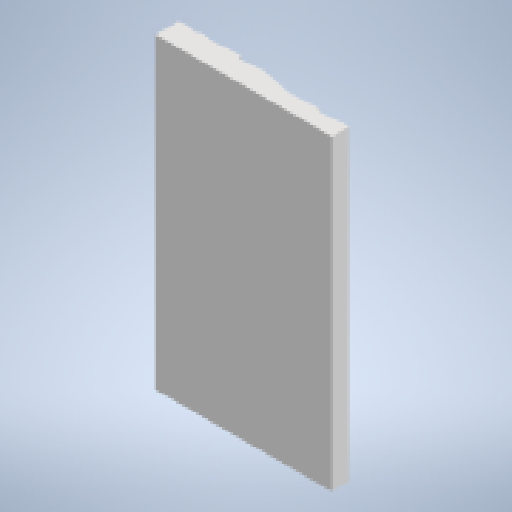
# Autodesk Inventor part: housingPlate
Saved by Autodesk Inventor 2023 (Build 270158000, 158)
## iProperties
Created: 2023-03-11
Part Number: housingPlate
Material: Generic
Document SubType Name: Modeling
Designer: shrey
Density: 1 g/cm^3
Appearance: Default
Author: shrey
Autodesk Inventor part; units mm, degrees
(part 1 of 2)
ref_plane "YZ Plane" through (0, 0, 0) normal (1, 0, 0) x (0, 1, 0)
ref_plane "XZ Plane" through (0, 0, 0) normal (0, 1, 0) x (-1, 0, 0)
ref_plane "XY Plane" through (0, 0, 0) normal (0, 0, 1) x (1, 0, 0)
sketch "Sketch1" plane through (0, 0, 0) normal (0, 0, 1) x (1, 0, 0)
  line L0 (58.171, 304.8) -> (58.171, -304.8) construction
  line L1 (-6.1102, -304.8) -> (58.171, -304.8) projected
  line L2 (-6.1102, 304.8) -> (-6.1102, -304.8) construction
  line L3 (58.171, 304.8) -> (-6.1102, 304.8) projected
  line L4 (-6.1102, 304.8) -> (-6.1102, -304.8) construction
  line L5 (-0.0002, -304.8) -> (-6.1102, -304.8) projected
  line L6 (-0.0002, 304.8) -> (-0.0002, -304.8) construction
  line L7 (-6.1102, 304.8) -> (-0.0002, 304.8) projected
  spline S0 degree 3 poles (-45.7965, -36.1769) (-45.6767, -35.9867) (-45.4969, -35.7016) (-45.2759, -35.3102) (-45.1171, -35.0129) (-44.9666, -34.7113) (-44.8248, -34.4054) (-44.6928, -34.0953) (-44.5714, -33.7808) (-44.4623, -33.4618) (-44.3664, -33.1385) (-44.3039, -32.8646) (-44.2588, -32.6445) (-44.2112, -32.4826) (-44.1468, -32.3266) (-44.0629, -32.1799) (-43.9744, -32.0702) (-43.8945, -31.991) (-43.8269, -31.9405) (-43.7577, -31.8921) (-43.6814, -31.856) (-43.6039, -31.8225) (-43.5218, -31.8027) (-43.4391, -31.786) (-43.3265, -31.782) (-43.1862, -31.7845) (-43.0458, -31.782) (-42.9332, -31.786) (-42.8505, -31.8027) (-42.7684, -31.8225) (-42.6909, -31.856) (-42.6146, -31.8921) (-42.5454, -31.9405) (-42.4778, -31.991) (-42.3979, -32.0702) (-42.3095, -32.1799) (-42.2255, -32.3266) (-42.1611, -32.4826) (-42.1135, -32.6445) (-42.0684, -32.8646) (-42.0059, -33.1385) (-41.91, -33.4618) (-41.8009, -33.7808) (-41.6795, -34.0953) (-41.5475, -34.4054) (-41.4057, -34.7113) (-41.2552, -35.0129) (-41.0964, -35.3102) (-40.8754, -35.7016) (-40.6956, -35.9867) (-40.5758, -36.1769) knots -1.0784 -1.0784 -1.0784 -1.0784 -1.010995 -0.977291 -0.943586 -0.909882 -0.876178 -0.842474 -0.80877 -0.775067 -0.741365 -0.707665 -0.690816 -0.67397 -0.657123 -0.640284 -0.623449 -0.615023 -0.606598 -0.598176 -0.589749 -0.581327 -0.572901 -0.564477 -0.556053 -0.5392 -0.522347 -0.513923 -0.505499 -0.497074 -0.488651 -0.480225 -0.471802 -0.463377 -0.454951 -0.438116 -0.421277 -0.40443 -0.387584 -0.370735 -0.337035 -0.303333 -0.26963 -0.235926 -0.202222 -0.168518 -0.134814 -0.101109 -0.067405 0 0 0 0 construction
  line L8 (-40.5758, -36.1769) -> (-39.5135, -36.1769) construction
  spline S1 degree 3 poles (-39.5135, -36.1769) (-39.3937, -35.9867) (-39.2139, -35.7016) (-38.9929, -35.3102) (-38.8341, -35.0129) (-38.6836, -34.7113) (-38.5418, -34.4054) (-38.4098, -34.0953) (-38.2884, -33.7808) (-38.1793, -33.4618) (-38.0834, -33.1385) (-38.0209, -32.8646) (-37.9758, -32.6445) (-37.9282, -32.4826) (-37.8638, -32.3266) (-37.7799, -32.1799) (-37.6914, -32.0702) (-37.6115, -31.991) (-37.5439, -31.9405) (-37.4747, -31.8921) (-37.3984, -31.856) (-37.3209, -31.8225) (-37.2388, -31.8027) (-37.1561, -31.786) (-37.0435, -31.782) (-36.9032, -31.7845) (-36.7628, -31.782) (-36.6502, -31.786) (-36.5675, -31.8027) (-36.4854, -31.8225) (-36.4079, -31.856) (-36.3316, -31.8921) (-36.2624, -31.9405) (-36.1948, -31.991) (-36.1149, -32.0702) (-36.0265, -32.1799) (-35.9425, -32.3266) (-35.8781, -32.4826) (-35.8305, -32.6445) (-35.7854, -32.8646) (-35.7229, -33.1385) (-35.627, -33.4618) (-35.5179, -33.7808) (-35.3965, -34.0953) (-35.2645, -34.4054) (-35.1227, -34.7113) (-34.9722, -35.0129) (-34.8134, -35.3102) (-34.5924, -35.7016) (-34.4126, -35.9867) (-34.2928, -36.1769) knots -1.0784 -1.0784 -1.0784 -1.0784 -1.010995 -0.977291 -0.943586 -0.909882 -0.876178 -0.842474 -0.80877 -0.775067 -0.741365 -0.707665 -0.690816 -0.67397 -0.657123 -0.640284 -0.623449 -0.615023 -0.606598 -0.598176 -0.589749 -0.581327 -0.572901 -0.564477 -0.556053 -0.5392 -0.522347 -0.513923 -0.505499 -0.497074 -0.488651 -0.480225 -0.471802 -0.463377 -0.454951 -0.438116 -0.421277 -0.40443 -0.387584 -0.370735 -0.337035 -0.303333 -0.26963 -0.235926 -0.202222 -0.168518 -0.134814 -0.101109 -0.067405 0 0 0 0 construction
  line L9 (-34.2928, -36.1769) -> (-33.2305, -36.1769) construction
  spline S2 degree 3 poles (-33.2305, -36.1769) (-33.1107, -35.9867) (-32.9309, -35.7016) (-32.7099, -35.3102) (-32.5511, -35.0129) (-32.4006, -34.7113) (-32.2588, -34.4054) (-32.1268, -34.0953) (-32.0054, -33.7808) (-31.8963, -33.4618) (-31.8004, -33.1385) (-31.7379, -32.8646) (-31.6928, -32.6445) (-31.6452, -32.4826) (-31.5808, -32.3266) (-31.4969, -32.1799) (-31.4084, -32.0702) (-31.3285, -31.991) (-31.2609, -31.9405) (-31.1917, -31.8921) (-31.1154, -31.856) (-31.0379, -31.8225) (-30.9558, -31.8027) (-30.8731, -31.786) (-30.7605, -31.782) (-30.6202, -31.7845) (-30.4798, -31.782) (-30.3672, -31.786) (-30.2845, -31.8027) (-30.2024, -31.8225) (-30.1249, -31.856) (-30.0486, -31.8921) (-29.9794, -31.9405) (-29.9118, -31.991) (-29.8319, -32.0702) (-29.7435, -32.1799) (-29.6595, -32.3266) (-29.5951, -32.4826) (-29.5475, -32.6445) (-29.5024, -32.8646) (-29.4399, -33.1385) (-29.344, -33.4618) (-29.2349, -33.7808) (-29.1135, -34.0953) (-28.9815, -34.4054) (-28.8397, -34.7113) (-28.6892, -35.0129) (-28.5304, -35.3102) (-28.3094, -35.7016) (-28.1296, -35.9867) (-28.0098, -36.1769) knots -1.0784 -1.0784 -1.0784 -1.0784 -1.010995 -0.977291 -0.943586 -0.909882 -0.876178 -0.842474 -0.80877 -0.775067 -0.741365 -0.707665 -0.690816 -0.67397 -0.657123 -0.640284 -0.623449 -0.615023 -0.606598 -0.598176 -0.589749 -0.581327 -0.572901 -0.564477 -0.556053 -0.5392 -0.522347 -0.513923 -0.505499 -0.497074 -0.488651 -0.480225 -0.471802 -0.463377 -0.454951 -0.438116 -0.421277 -0.40443 -0.387584 -0.370735 -0.337035 -0.303333 -0.26963 -0.235926 -0.202222 -0.168518 -0.134814 -0.101109 -0.067405 0 0 0 0 construction
  line L10 (-28.0098, -36.1769) -> (-26.9475, -36.1769) construction
  spline S3 degree 3 poles (-26.9475, -36.1769) (-26.8277, -35.9867) (-26.6479, -35.7016) (-26.4269, -35.3102) (-26.2681, -35.0129) (-26.1176, -34.7113) (-25.9758, -34.4054) (-25.8438, -34.0953) (-25.7224, -33.7808) (-25.6133, -33.4618) (-25.5174, -33.1385) (-25.4549, -32.8646) (-25.4098, -32.6445) (-25.3622, -32.4826) (-25.2978, -32.3266) (-25.2139, -32.1799) (-25.1254, -32.0702) (-25.0455, -31.991) (-24.9779, -31.9405) (-24.9087, -31.8921) (-24.8324, -31.856) (-24.7549, -31.8225) (-24.6728, -31.8027) (-24.5901, -31.786) (-24.4775, -31.782) (-24.3372, -31.7845) (-24.1968, -31.782) (-24.0842, -31.786) (-24.0015, -31.8027) (-23.9194, -31.8225) (-23.8419, -31.856) (-23.7656, -31.8921) (-23.6964, -31.9405) (-23.6288, -31.991) (-23.5489, -32.0702) (-23.4605, -32.1799) (-23.3765, -32.3266) (-23.3121, -32.4826) (-23.2645, -32.6445) (-23.2194, -32.8646) (-23.1569, -33.1385) (-23.061, -33.4618) (-22.9519, -33.7808) (-22.8305, -34.0953) (-22.6985, -34.4054) (-22.5567, -34.7113) (-22.4062, -35.0129) (-22.2474, -35.3102) (-22.0264, -35.7016) (-21.8466, -35.9867) (-21.7268, -36.1769) knots -1.0784 -1.0784 -1.0784 -1.0784 -1.010995 -0.977291 -0.943586 -0.909882 -0.876178 -0.842474 -0.80877 -0.775067 -0.741365 -0.707665 -0.690816 -0.67397 -0.657123 -0.640284 -0.623449 -0.615023 -0.606598 -0.598176 -0.589749 -0.581327 -0.572901 -0.564477 -0.556053 -0.5392 -0.522347 -0.513923 -0.505499 -0.497074 -0.488651 -0.480225 -0.471802 -0.463377 -0.454951 -0.438116 -0.421277 -0.40443 -0.387584 -0.370735 -0.337035 -0.303333 -0.26963 -0.235926 -0.202222 -0.168518 -0.134814 -0.101109 -0.067405 0 0 0 0 construction
  line L11 (-21.7268, -36.1769) -> (-20.6645, -36.1769) construction
  spline S4 degree 3 poles (-20.6645, -36.1769) (-20.5447, -35.9867) (-20.3649, -35.7016) (-20.1439, -35.3102) (-19.9851, -35.0129) (-19.8346, -34.7113) (-19.6928, -34.4054) (-19.5608, -34.0953) (-19.4394, -33.7808) (-19.3303, -33.4618) (-19.2344, -33.1385) (-19.1719, -32.8646) (-19.1268, -32.6445) (-19.0792, -32.4826) (-19.0148, -32.3266) (-18.9309, -32.1799) (-18.8424, -32.0702) (-18.7625, -31.991) (-18.6949, -31.9405) (-18.6257, -31.8921) (-18.5494, -31.856) (-18.4719, -31.8225) (-18.3898, -31.8027) (-18.3071, -31.786) (-18.1945, -31.782) (-18.0542, -31.7845) (-17.9138, -31.782) (-17.8012, -31.786) (-17.7185, -31.8027) (-17.6364, -31.8225) (-17.5589, -31.856) (-17.4826, -31.8921) (-17.4134, -31.9405) (-17.3458, -31.991) (-17.2659, -32.0702) (-17.1775, -32.1799) (-17.0935, -32.3266) (-17.0291, -32.4826) (-16.9815, -32.6445) (-16.9364, -32.8646) (-16.8739, -33.1385) (-16.778, -33.4618) (-16.6689, -33.7808) (-16.5475, -34.0953) (-16.4155, -34.4054) (-16.2737, -34.7113) (-16.1232, -35.0129) (-15.9644, -35.3102) (-15.7434, -35.7016) (-15.5636, -35.9867) (-15.4438, -36.1769) knots -1.0784 -1.0784 -1.0784 -1.0784 -1.010995 -0.977291 -0.943586 -0.909882 -0.876178 -0.842474 -0.80877 -0.775067 -0.741365 -0.707665 -0.690816 -0.67397 -0.657123 -0.640284 -0.623449 -0.615023 -0.606598 -0.598176 -0.589749 -0.581327 -0.572901 -0.564477 -0.556053 -0.5392 -0.522347 -0.513923 -0.505499 -0.497074 -0.488651 -0.480225 -0.471802 -0.463377 -0.454951 -0.438116 -0.421277 -0.40443 -0.387584 -0.370735 -0.337035 -0.303333 -0.26963 -0.235926 -0.202222 -0.168518 -0.134814 -0.101109 -0.067405 0 0 0 0 construction
  line L12 (-15.4438, -36.1769) -> (-14.3815, -36.1769) construction
  spline S5 degree 3 poles (-14.3815, -36.1769) (-14.2617, -35.9867) (-14.0819, -35.7016) (-13.8609, -35.3102) (-13.7021, -35.0129) (-13.5516, -34.7113) (-13.4098, -34.4054) (-13.2778, -34.0953) (-13.1564, -33.7808) (-13.0473, -33.4618) (-12.9514, -33.1385) (-12.8889, -32.8646) (-12.8438, -32.6445) (-12.7962, -32.4826) (-12.7318, -32.3266) (-12.6479, -32.1799) (-12.5594, -32.0702) (-12.4795, -31.991) (-12.4119, -31.9405) (-12.3427, -31.8921) (-12.2664, -31.856) (-12.1889, -31.8225) (-12.1068, -31.8027) (-12.0241, -31.786) (-11.9115, -31.782) (-11.7712, -31.7845) (-11.6308, -31.782) (-11.5182, -31.786) (-11.4355, -31.8027) (-11.3534, -31.8225) (-11.2759, -31.856) (-11.1996, -31.8921) (-11.1304, -31.9405) (-11.0628, -31.991) (-10.9829, -32.0702) (-10.8945, -32.1799) (-10.8105, -32.3266) (-10.7461, -32.4826) (-10.6985, -32.6445) (-10.6534, -32.8646) (-10.5909, -33.1385) (-10.495, -33.4618) (-10.3859, -33.7808) (-10.2645, -34.0953) (-10.1325, -34.4054) (-9.9907, -34.7113) (-9.8402, -35.0129) (-9.6814, -35.3102) (-9.4604, -35.7016) (-9.2806, -35.9867) (-9.1608, -36.1769) knots -1.0784 -1.0784 -1.0784 -1.0784 -1.010995 -0.977291 -0.943586 -0.909882 -0.876178 -0.842474 -0.80877 -0.775067 -0.741365 -0.707665 -0.690816 -0.67397 -0.657123 -0.640284 -0.623449 -0.615023 -0.606598 -0.598176 -0.589749 -0.581327 -0.572901 -0.564477 -0.556053 -0.5392 -0.522347 -0.513923 -0.505499 -0.497074 -0.488651 -0.480225 -0.471802 -0.463377 -0.454951 -0.438116 -0.421277 -0.40443 -0.387584 -0.370735 -0.337035 -0.303333 -0.26963 -0.235926 -0.202222 -0.168518 -0.134814 -0.101109 -0.067405 0 0 0 0 construction
  line L13 (-9.1608, -36.1769) -> (-8.0985, -36.1769) construction
  spline S6 degree 3 poles (-8.0985, -36.1769) (-7.9787, -35.9867) (-7.7989, -35.7016) (-7.5779, -35.3102) (-7.4191, -35.0129) (-7.2686, -34.7113) (-7.1268, -34.4054) (-6.9948, -34.0953) (-6.8734, -33.7808) (-6.7643, -33.4618) (-6.6684, -33.1385) (-6.6059, -32.8646) (-6.5608, -32.6445) (-6.5132, -32.4826) (-6.4488, -32.3266) (-6.3649, -32.1799) (-6.2764, -32.0702) (-6.1965, -31.991) (-6.1289, -31.9405) (-6.0597, -31.8921) (-5.9834, -31.856) (-5.9059, -31.8225) (-5.8238, -31.8027) (-5.7411, -31.786) (-5.6285, -31.782) (-5.4882, -31.7845) (-5.3478, -31.782) (-5.2352, -31.786) (-5.1525, -31.8027) (-5.0704, -31.8225) (-4.9929, -31.856) (-4.9166, -31.8921) (-4.8474, -31.9405) (-4.7798, -31.991) (-4.6999, -32.0702) (-4.6115, -32.1799) (-4.5275, -32.3266) (-4.4631, -32.4826) (-4.4155, -32.6445) (-4.3704, -32.8646) (-4.3079, -33.1385) (-4.212, -33.4618) (-4.1029, -33.7808) (-3.9815, -34.0953) (-3.8495, -34.4054) (-3.7077, -34.7113) (-3.5572, -35.0129) (-3.3984, -35.3102) (-3.1774, -35.7016) (-2.9976, -35.9867) (-2.8778, -36.1769) knots -1.0784 -1.0784 -1.0784 -1.0784 -1.010995 -0.977291 -0.943586 -0.909882 -0.876178 -0.842474 -0.80877 -0.775067 -0.741365 -0.707665 -0.690816 -0.67397 -0.657123 -0.640284 -0.623449 -0.615023 -0.606598 -0.598176 -0.589749 -0.581327 -0.572901 -0.564477 -0.556053 -0.5392 -0.522347 -0.513923 -0.505499 -0.497074 -0.488651 -0.480225 -0.471802 -0.463377 -0.454951 -0.438116 -0.421277 -0.40443 -0.387584 -0.370735 -0.337035 -0.303333 -0.26963 -0.235926 -0.202222 -0.168518 -0.134814 -0.101109 -0.067405 0 0 0 0 construction
  line L14 (-2.8778, -36.1769) -> (-1.8155, -36.1769) construction
  spline S7 degree 3 poles (-1.8155, -36.1769) (-1.6957, -35.9867) (-1.5159, -35.7016) (-1.2949, -35.3102) (-1.1361, -35.0129) (-0.9856, -34.7113) (-0.8438, -34.4054) (-0.7118, -34.0953) (-0.5904, -33.7808) (-0.4813, -33.4618) (-0.3854, -33.1385) (-0.3229, -32.8646) (-0.2778, -32.6445) (-0.2302, -32.4826) (-0.1658, -32.3266) (-0.0819, -32.1799) (0.0066, -32.0702) (0.0865, -31.991) (0.1541, -31.9405) (0.2233, -31.8921) (0.2996, -31.856) (0.3771, -31.8225) (0.4592, -31.8027) (0.5419, -31.786) (0.6545, -31.782) (0.7948, -31.7845) (0.9352, -31.782) (1.0478, -31.786) (1.1305, -31.8027) (1.2126, -31.8225) (1.2901, -31.856) (1.3664, -31.8921) (1.4356, -31.9405) (1.5032, -31.991) (1.5831, -32.0702) (1.6715, -32.1799) (1.7555, -32.3266) (1.8199, -32.4826) (1.8675, -32.6445) (1.9126, -32.8646) (1.9751, -33.1385) (2.071, -33.4618) (2.1801, -33.7808) (2.3015, -34.0953) (2.4335, -34.4054) (2.5753, -34.7113) (2.7258, -35.0129) (2.8846, -35.3102) (3.1056, -35.7016) (3.2854, -35.9867) (3.4052, -36.1769) knots -1.0784 -1.0784 -1.0784 -1.0784 -1.010995 -0.977291 -0.943586 -0.909882 -0.876178 -0.842474 -0.80877 -0.775067 -0.741365 -0.707665 -0.690816 -0.67397 -0.657123 -0.640284 -0.623449 -0.615023 -0.606598 -0.598176 -0.589749 -0.581327 -0.572901 -0.564477 -0.556053 -0.5392 -0.522347 -0.513923 -0.505499 -0.497074 -0.488651 -0.480225 -0.471802 -0.463377 -0.454951 -0.438116 -0.421277 -0.40443 -0.387584 -0.370735 -0.337035 -0.303333 -0.26963 -0.235926 -0.202222 -0.168518 -0.134814 -0.101109 -0.067405 0 0 0 0 construction
  line L15 (3.4052, -36.1769) -> (4.4675, -36.1769) construction
  spline S8 degree 3 poles (4.4675, -36.1769) (4.5873, -35.9867) (4.7671, -35.7016) (4.9881, -35.3102) (5.1469, -35.0129) (5.2974, -34.7113) (5.4392, -34.4054) (5.5712, -34.0953) (5.6926, -33.7808) (5.8017, -33.4618) (5.8976, -33.1385) (5.9601, -32.8646) (6.0052, -32.6445) (6.0528, -32.4826) (6.1172, -32.3266) (6.2011, -32.1799) (6.2896, -32.0702) (6.3695, -31.991) (6.4371, -31.9405) (6.5063, -31.8921) (6.5826, -31.856) (6.6601, -31.8225) (6.7422, -31.8027) (6.8249, -31.786) (6.9375, -31.782) (7.0778, -31.7845) (7.2182, -31.782) (7.3308, -31.786) (7.4135, -31.8027) (7.4956, -31.8225) (7.5731, -31.856) (7.6494, -31.8921) (7.7186, -31.9405) (7.7862, -31.991) (7.8661, -32.0702) (7.9545, -32.1799) (8.0385, -32.3266) (8.1029, -32.4826) (8.1505, -32.6445) (8.1956, -32.8646) (8.2581, -33.1385) (8.354, -33.4618) (8.4631, -33.7808) (8.5845, -34.0953) (8.7165, -34.4054) (8.8583, -34.7113) (9.0088, -35.0129) (9.1676, -35.3102) (9.3886, -35.7016) (9.5684, -35.9867) (9.6882, -36.1769) knots -1.0784 -1.0784 -1.0784 -1.0784 -1.010995 -0.977291 -0.943586 -0.909882 -0.876178 -0.842474 -0.80877 -0.775067 -0.741365 -0.707665 -0.690816 -0.67397 -0.657123 -0.640284 -0.623449 -0.615023 -0.606598 -0.598176 -0.589749 -0.581327 -0.572901 -0.564477 -0.556053 -0.5392 -0.522347 -0.513923 -0.505499 -0.497074 -0.488651 -0.480225 -0.471802 -0.463377 -0.454951 -0.438116 -0.421277 -0.40443 -0.387584 -0.370735 -0.337035 -0.303333 -0.26963 -0.235926 -0.202222 -0.168518 -0.134814 -0.101109 -0.067405 0 0 0 0 construction
  line L16 (9.6882, -36.1769) -> (10.7505, -36.1769) construction
  spline S9 degree 3 poles (10.7505, -36.1769) (10.8703, -35.9867) (11.0501, -35.7016) (11.2711, -35.3102) (11.4299, -35.0129) (11.5804, -34.7113) (11.7222, -34.4054) (11.8542, -34.0953) (11.9756, -33.7808) (12.0847, -33.4618) (12.1806, -33.1385) (12.2431, -32.8646) (12.2882, -32.6445) (12.3358, -32.4826) (12.4002, -32.3266) (12.4841, -32.1799) (12.5726, -32.0702) (12.6525, -31.991) (12.7201, -31.9405) (12.7893, -31.8921) (12.8656, -31.856) (12.9431, -31.8225) (13.0252, -31.8027) (13.1079, -31.786) (13.2205, -31.782) (13.3608, -31.7845) (13.5012, -31.782) (13.6138, -31.786) (13.6965, -31.8027) (13.7786, -31.8225) (13.8561, -31.856) (13.9324, -31.8921) (14.0016, -31.9405) (14.0692, -31.991) (14.1491, -32.0702) (14.2375, -32.1799) (14.3215, -32.3266) (14.3859, -32.4826) (14.4335, -32.6445) (14.4786, -32.8646) (14.5411, -33.1385) (14.637, -33.4618) (14.7461, -33.7808) (14.8675, -34.0953) (14.9995, -34.4054) (15.1413, -34.7113) (15.2918, -35.0129) (15.4506, -35.3102) (15.6716, -35.7016) (15.8514, -35.9867) (15.9712, -36.1769) knots -1.0784 -1.0784 -1.0784 -1.0784 -1.010995 -0.977291 -0.943586 -0.909882 -0.876178 -0.842474 -0.80877 -0.775067 -0.741365 -0.707665 -0.690816 -0.67397 -0.657123 -0.640284 -0.623449 -0.615023 -0.606598 -0.598176 -0.589749 -0.581327 -0.572901 -0.564477 -0.556053 -0.5392 -0.522347 -0.513923 -0.505499 -0.497074 -0.488651 -0.480225 -0.471802 -0.463377 -0.454951 -0.438116 -0.421277 -0.40443 -0.387584 -0.370735 -0.337035 -0.303333 -0.26963 -0.235926 -0.202222 -0.168518 -0.134814 -0.101109 -0.067405 0 0 0 0 construction
  line L17 (15.9712, -36.1769) -> (17.0335, -36.1769) construction
  spline S10 degree 3 poles (17.0335, -36.1769) (17.1533, -35.9867) (17.3331, -35.7016) (17.5541, -35.3102) (17.7129, -35.0129) (17.8634, -34.7113) (18.0052, -34.4054) (18.1372, -34.0953) (18.2586, -33.7808) (18.3677, -33.4618) (18.4636, -33.1385) (18.5261, -32.8646) (18.5712, -32.6445) (18.6188, -32.4826) (18.6832, -32.3266) (18.7671, -32.1799) (18.8556, -32.0702) (18.9355, -31.991) (19.0031, -31.9405) (19.0723, -31.8921) (19.1486, -31.856) (19.2261, -31.8225) (19.3082, -31.8027) (19.3909, -31.786) (19.5035, -31.782) (19.6438, -31.7845) (19.7842, -31.782) (19.8968, -31.786) (19.9795, -31.8027) (20.0616, -31.8225) (20.1391, -31.856) (20.2154, -31.8921) (20.2846, -31.9405) (20.3522, -31.991) (20.4321, -32.0702) (20.5205, -32.1799) (20.6045, -32.3266) (20.6689, -32.4826) (20.7165, -32.6445) (20.7616, -32.8646) (20.8241, -33.1385) (20.92, -33.4618) (21.0291, -33.7808) (21.1505, -34.0953) (21.2825, -34.4054) (21.4243, -34.7113) (21.5748, -35.0129) (21.7336, -35.3102) (21.9546, -35.7016) (22.1344, -35.9867) (22.2542, -36.1769) knots -1.0784 -1.0784 -1.0784 -1.0784 -1.010995 -0.977291 -0.943586 -0.909882 -0.876178 -0.842474 -0.80877 -0.775067 -0.741365 -0.707665 -0.690816 -0.67397 -0.657123 -0.640284 -0.623449 -0.615023 -0.606598 -0.598176 -0.589749 -0.581327 -0.572901 -0.564477 -0.556053 -0.5392 -0.522347 -0.513923 -0.505499 -0.497074 -0.488651 -0.480225 -0.471802 -0.463377 -0.454951 -0.438116 -0.421277 -0.40443 -0.387584 -0.370735 -0.337035 -0.303333 -0.26963 -0.235926 -0.202222 -0.168518 -0.134814 -0.101109 -0.067405 0 0 0 0 construction
  line L18 (22.2542, -36.1769) -> (23.3165, -36.1769) construction
  spline S11 degree 3 poles (23.3165, -36.1769) (23.4363, -35.9867) (23.6161, -35.7016) (23.8371, -35.3102) (23.9959, -35.0129) (24.1464, -34.7113) (24.2882, -34.4054) (24.4202, -34.0953) (24.5416, -33.7808) (24.6507, -33.4618) (24.7466, -33.1385) (24.8091, -32.8646) (24.8542, -32.6445) (24.9018, -32.4826) (24.9662, -32.3266) (25.0501, -32.1799) (25.1386, -32.0702) (25.2185, -31.991) (25.2861, -31.9405) (25.3553, -31.8921) (25.4316, -31.856) (25.5091, -31.8225) (25.5912, -31.8027) (25.6739, -31.786) (25.7865, -31.782) (25.9268, -31.7845) (26.0672, -31.782) (26.1798, -31.786) (26.2625, -31.8027) (26.3446, -31.8225) (26.4221, -31.856) (26.4984, -31.8921) (26.5676, -31.9405) (26.6352, -31.991) (26.7151, -32.0702) (26.8035, -32.1799) (26.8875, -32.3266) (26.9519, -32.4826) (26.9995, -32.6445) (27.0446, -32.8646) (27.1071, -33.1385) (27.203, -33.4618) (27.3121, -33.7808) (27.4335, -34.0953) (27.5655, -34.4054) (27.7073, -34.7113) (27.8578, -35.0129) (28.0166, -35.3102) (28.2376, -35.7016) (28.4174, -35.9867) (28.5372, -36.1769) knots -1.0784 -1.0784 -1.0784 -1.0784 -1.010995 -0.977291 -0.943586 -0.909882 -0.876178 -0.842474 -0.80877 -0.775067 -0.741365 -0.707665 -0.690816 -0.67397 -0.657123 -0.640284 -0.623449 -0.615023 -0.606598 -0.598176 -0.589749 -0.581327 -0.572901 -0.564477 -0.556053 -0.5392 -0.522347 -0.513923 -0.505499 -0.497074 -0.488651 -0.480225 -0.471802 -0.463377 -0.454951 -0.438116 -0.421277 -0.40443 -0.387584 -0.370735 -0.337035 -0.303333 -0.26963 -0.235926 -0.202222 -0.168518 -0.134814 -0.101109 -0.067405 0 0 0 0 construction
  line L19 (28.5372, -36.1769) -> (29.5995, -36.1769) construction
  spline S12 degree 3 poles (29.5995, -36.1769) (29.7193, -35.9867) (29.8991, -35.7016) (30.1201, -35.3102) (30.2789, -35.0129) (30.4294, -34.7113) (30.5712, -34.4054) (30.7032, -34.0953) (30.8246, -33.7808) (30.9337, -33.4618) (31.0296, -33.1385) (31.0921, -32.8646) (31.1372, -32.6445) (31.1848, -32.4826) (31.2492, -32.3266) (31.3331, -32.1799) (31.4216, -32.0702) (31.5015, -31.991) (31.5691, -31.9405) (31.6383, -31.8921) (31.7146, -31.856) (31.7921, -31.8225) (31.8742, -31.8027) (31.9569, -31.786) (32.0695, -31.782) (32.2098, -31.7845) (32.3502, -31.782) (32.4628, -31.786) (32.5455, -31.8027) (32.6276, -31.8225) (32.7051, -31.856) (32.7814, -31.8921) (32.8506, -31.9405) (32.9182, -31.991) (32.9981, -32.0702) (33.0865, -32.1799) (33.1705, -32.3266) (33.2349, -32.4826) (33.2825, -32.6445) (33.3276, -32.8646) (33.3901, -33.1385) (33.486, -33.4618) (33.5951, -33.7808) (33.7165, -34.0953) (33.8485, -34.4054) (33.9903, -34.7113) (34.1408, -35.0129) (34.2996, -35.3102) (34.5206, -35.7016) (34.7004, -35.9867) (34.8202, -36.1769) knots -1.0784 -1.0784 -1.0784 -1.0784 -1.010995 -0.977291 -0.943586 -0.909882 -0.876178 -0.842474 -0.80877 -0.775067 -0.741365 -0.707665 -0.690816 -0.67397 -0.657123 -0.640284 -0.623449 -0.615023 -0.606598 -0.598176 -0.589749 -0.581327 -0.572901 -0.564477 -0.556053 -0.5392 -0.522347 -0.513923 -0.505499 -0.497074 -0.488651 -0.480225 -0.471802 -0.463377 -0.454951 -0.438116 -0.421277 -0.40443 -0.387584 -0.370735 -0.337035 -0.303333 -0.26963 -0.235926 -0.202222 -0.168518 -0.134814 -0.101109 -0.067405 0 0 0 0 construction
  line L20 (34.8202, -36.1769) -> (35.8825, -36.1769) construction
  spline S13 degree 3 poles (35.8825, -36.1769) (36.0023, -35.9867) (36.1821, -35.7016) (36.4031, -35.3102) (36.5619, -35.0129) (36.7124, -34.7113) (36.8542, -34.4054) (36.9862, -34.0953) (37.1076, -33.7808) (37.2167, -33.4618) (37.3126, -33.1385) (37.3751, -32.8646) (37.4202, -32.6445) (37.4678, -32.4826) (37.5322, -32.3266) (37.6161, -32.1799) (37.7046, -32.0702) (37.7845, -31.991) (37.8521, -31.9405) (37.9213, -31.8921) (37.9976, -31.856) (38.0751, -31.8225) (38.1572, -31.8027) (38.2399, -31.786) (38.3525, -31.782) (38.4928, -31.7845) (38.6332, -31.782) (38.7458, -31.786) (38.8285, -31.8027) (38.9106, -31.8225) (38.9881, -31.856) (39.0644, -31.8921) (39.1336, -31.9405) (39.2012, -31.991) (39.2811, -32.0702) (39.3695, -32.1799) (39.4535, -32.3266) (39.5179, -32.4826) (39.5655, -32.6445) (39.6106, -32.8646) (39.6731, -33.1385) (39.769, -33.4618) (39.8781, -33.7808) (39.9995, -34.0953) (40.1315, -34.4054) (40.2733, -34.7113) (40.4238, -35.0129) (40.5826, -35.3102) (40.8036, -35.7016) (40.9834, -35.9867) (41.1032, -36.1769) knots -1.0784 -1.0784 -1.0784 -1.0784 -1.010995 -0.977291 -0.943586 -0.909882 -0.876178 -0.842474 -0.80877 -0.775067 -0.741365 -0.707665 -0.690816 -0.67397 -0.657123 -0.640284 -0.623449 -0.615023 -0.606598 -0.598176 -0.589749 -0.581327 -0.572901 -0.564477 -0.556053 -0.5392 -0.522347 -0.513923 -0.505499 -0.497074 -0.488651 -0.480225 -0.471802 -0.463377 -0.454951 -0.438116 -0.421277 -0.40443 -0.387584 -0.370735 -0.337035 -0.303333 -0.26963 -0.235926 -0.202222 -0.168518 -0.134814 -0.101109 -0.067405 0 0 0 0 construction
  line L21 (41.1032, -36.1769) -> (42.1655, -36.1769) construction
  spline S14 degree 3 poles (42.1655, -36.1769) (42.2853, -35.9867) (42.4651, -35.7016) (42.6861, -35.3102) (42.8449, -35.0129) (42.9954, -34.7113) (43.1372, -34.4054) (43.2692, -34.0953) (43.3906, -33.7808) (43.4997, -33.4618) (43.5956, -33.1385) (43.6581, -32.8646) (43.7032, -32.6445) (43.7508, -32.4826) (43.8152, -32.3266) (43.8991, -32.1799) (43.9876, -32.0702) (44.0675, -31.991) (44.1351, -31.9405) (44.2043, -31.8921) (44.2806, -31.856) (44.3581, -31.8225) (44.4402, -31.8027) (44.5229, -31.786) (44.6355, -31.782) (44.7758, -31.7845) (44.9162, -31.782) (45.0288, -31.786) (45.1115, -31.8027) (45.1936, -31.8225) (45.2711, -31.856) (45.3474, -31.8921) (45.4166, -31.9405) (45.4842, -31.991) (45.5641, -32.0702) (45.6525, -32.1799) (45.7365, -32.3266) (45.8009, -32.4826) (45.8485, -32.6445) (45.8936, -32.8646) (45.9561, -33.1385) (46.052, -33.4618) (46.1611, -33.7808) (46.2825, -34.0953) (46.4145, -34.4054) (46.5563, -34.7113) (46.7068, -35.0129) (46.8656, -35.3102) (47.0866, -35.7016) (47.2664, -35.9867) (47.3862, -36.1769) knots -1.0784 -1.0784 -1.0784 -1.0784 -1.010995 -0.977291 -0.943586 -0.909882 -0.876178 -0.842474 -0.80877 -0.775067 -0.741365 -0.707665 -0.690816 -0.67397 -0.657123 -0.640284 -0.623449 -0.615023 -0.606598 -0.598176 -0.589749 -0.581327 -0.572901 -0.564477 -0.556053 -0.5392 -0.522347 -0.513923 -0.505499 -0.497074 -0.488651 -0.480225 -0.471802 -0.463377 -0.454951 -0.438116 -0.421277 -0.40443 -0.387584 -0.370735 -0.337035 -0.303333 -0.26963 -0.235926 -0.202222 -0.168518 -0.134814 -0.101109 -0.067405 0 0 0 0 construction
  line L22 (47.3862, -36.1769) -> (48.4485, -36.1769) construction
  spline S15 degree 3 poles (48.4485, -36.1769) (48.7016, -35.7753) (49.2786, -34.8601) (50.003, -32.8691) (49.9556, -32.5218) (50.283, -32.0392) (50.3898, -31.959) (50.4933, -31.8895) (50.5898, -31.8295) (50.8834, -31.7709) (51.0193, -31.7835) (51.2695, -31.7827) (51.3802, -31.7851) (51.6043, -31.8754) (51.698, -31.9358) (51.8372, -32.0518) (51.8987, -32.1341) (52.0075, -32.2925) (52.0634, -32.4204) (52.16, -32.737) (52.1755, -32.898) (52.6522, -34.6151) (53.4935, -35.8981) (53.6692, -36.1769) knots 0 0 0 0 0.142394 0.142394 0.262557 0.262557 0.314666 0.314666 0.34653 0.34653 0.372217 0.372217 0.394622 0.394622 0.411062 0.411062 0.432958 0.432958 0.48678 0.48678 0.562983 0.562983 0.900876 0.900876 0.900876 0.900876 construction
  line L23 (53.6692, -36.1769) -> (53.6692, -26.7835) construction
  line L24 (53.6692, -26.7835) -> (-46.3308, -26.7835) construction
  line L25 (-46.3308, -26.7835) -> (-46.3308, -36.1769) construction
  line L26 (-46.3308, -36.1769) -> (-45.7965, -36.1769) construction
  arc A0 (11.4363, -73.1689) -> (34.3606, -89.8244) centre (35.3606, -64.344) ccw construction
  line L27 (11.4363, -73.1689) -> (23.271, -69.3236) construction
  arc A1 (23.271, -69.3236) -> (34.3606, -77.3807) centre (35.3606, -64.344) ccw construction
  line L28 (34.3606, -77.3807) -> (34.3606, -89.8244) construction
  line L29 (59.9029, -71.2668) -> (48.0682, -67.4215) construction
  arc A2 (48.0682, -67.4215) -> (43.8324, -54.3849) centre (35.3606, -64.344) ccw construction
  line L30 (43.8324, -54.3849) -> (51.1466, -44.3177) construction
  arc A3 (59.9029, -71.2668) -> (51.1466, -44.3177) centre (35.3606, -64.344) ccw construction
  line L31 (19.5746, -44.3177) -> (26.8888, -54.3849) construction
  arc A4 (26.8888, -54.3849) -> (22.6529, -67.4215) centre (35.3606, -64.344) ccw construction
  line L32 (22.6529, -67.4215) -> (10.8183, -71.2668) construction
  arc A5 (19.5746, -44.3177) -> (10.8183, -71.2668) centre (35.3606, -64.344) ccw construction
  circle A6 centre (35.3606, -64.344) radius 11.075 construction
  line L33 (49.5286, -43.1422) -> (42.2143, -53.2093) construction
  arc A7 (42.2143, -53.2093) -> (28.5068, -53.2093) centre (35.3606, -64.344) ccw construction
  line L34 (28.5068, -53.2093) -> (21.1926, -43.1422) construction
  arc A8 (49.5286, -43.1422) -> (21.1926, -43.1422) centre (35.3606, -64.344) ccw construction
  line L35 (36.3606, -89.8244) -> (36.3606, -77.3807) construction
  arc A9 (36.3606, -77.3807) -> (47.4502, -69.3236) centre (35.3606, -64.344) ccw construction
  line L36 (47.4502, -69.3236) -> (59.2848, -73.1689) construction
  arc A10 (36.3606, -89.8244) -> (59.2848, -73.1689) centre (35.3606, -64.344) ccw construction
  spline S16 degree 3 poles (39.4382, -96.0832) (39.5159, -95.8723) (39.6325, -95.556) (39.7673, -95.1272) (39.8609, -94.8034) (39.9454, -94.477) (40.0204, -94.1484) (40.0851, -93.8176) (40.1384, -93.4847) (40.1788, -93.15) (40.2054, -92.8139) (40.2096, -92.533) (40.2079, -92.3083) (40.2209, -92.14) (40.2514, -91.974) (40.303, -91.813) (40.3668, -91.6874) (40.4284, -91.5933) (40.484, -91.5299) (40.5417, -91.4681) (40.6088, -91.4169) (40.6776, -91.368) (40.7538, -91.3316) (40.8313, -91.2981) (40.9405, -91.2707) (41.0784, -91.2441) (41.2151, -91.2124) (41.326, -91.1929) (41.4105, -91.192) (41.4949, -91.1943) (41.5776, -91.211) (41.6598, -91.2305) (41.7375, -91.2634) (41.8141, -91.2988) (41.9088, -91.3596) (42.0181, -91.4485) (42.1307, -91.5746) (42.2261, -91.7138) (42.3064, -91.8622) (42.3963, -92.0682) (42.5143, -92.3231) (42.6754, -92.6194) (42.8484, -92.9087) (43.0325, -93.1911) (43.2262, -93.467) (43.4284, -93.7367) (43.6383, -94.0005) (43.8555, -94.2583) (44.153, -94.5951) (44.3882, -94.8367) (44.5449, -94.9977) knots -1.0784 -1.0784 -1.0784 -1.0784 -1.010995 -0.977291 -0.943586 -0.909882 -0.876178 -0.842474 -0.80877 -0.775067 -0.741365 -0.707665 -0.690816 -0.67397 -0.657123 -0.640284 -0.623449 -0.615023 -0.606598 -0.598176 -0.589749 -0.581327 -0.572901 -0.564477 -0.556053 -0.5392 -0.522347 -0.513923 -0.505499 -0.497074 -0.488651 -0.480225 -0.471802 -0.463377 -0.454951 -0.438116 -0.421277 -0.40443 -0.387584 -0.370735 -0.337035 -0.303333 -0.26963 -0.235926 -0.202222 -0.168518 -0.134814 -0.101109 -0.067405 0 0 0 0 construction
  arc A11 (44.5449, -94.9977) -> (45.9481, -94.5418) centre (35.3606, -64.344) ccw construction
  spline S17 degree 3 poles (45.9481, -94.5418) (45.9802, -94.3194) (46.0285, -93.9857) (46.0712, -93.5383) (46.0954, -93.2021) (46.1102, -92.8653) (46.1153, -92.5283) (46.1097, -92.1912) (46.0927, -91.8545) (46.0626, -91.5188) (46.0188, -91.1844) (45.9644, -90.9088) (45.9161, -90.6894) (45.8938, -90.5221) (45.8891, -90.3534) (45.9061, -90.1852) (45.9424, -90.0491) (45.9831, -89.9442) (46.0243, -89.8706) (46.0679, -89.7982) (46.1229, -89.7342) (46.1801, -89.672) (46.247, -89.6205) (46.3158, -89.5716) (46.417, -89.5222) (46.5463, -89.4675) (46.6734, -89.408) (46.7779, -89.3659) (46.8603, -89.3475) (46.9433, -89.3322) (47.0277, -89.3313) (47.1121, -89.3333) (47.195, -89.3493) (47.2773, -89.368) (47.3825, -89.4078) (47.508, -89.472) (47.6443, -89.5719) (47.7666, -89.6883) (47.876, -89.8168) (48.0067, -89.9995) (48.1752, -90.2243) (48.3943, -90.4806) (48.6237, -90.7277) (48.8625, -90.9656) (49.1093, -91.1953) (49.3632, -91.417) (49.6233, -91.6314) (49.8893, -91.8384) (50.2504, -92.106) (50.5307, -92.2934) (50.7175, -92.4183) knots -1.0784 -1.0784 -1.0784 -1.0784 -1.010995 -0.977291 -0.943586 -0.909882 -0.876178 -0.842474 -0.80877 -0.775067 -0.741365 -0.707665 -0.690816 -0.67397 -0.657123 -0.640284 -0.623449 -0.615023 -0.606598 -0.598176 -0.589749 -0.581327 -0.572901 -0.564477 -0.556053 -0.5392 -0.522347 -0.513923 -0.505499 -0.497074 -0.488651 -0.480225 -0.471802 -0.463377 -0.454951 -0.438116 -0.421277 -0.40443 -0.387584 -0.370735 -0.337035 -0.303333 -0.26963 -0.235926 -0.202222 -0.168518 -0.134814 -0.101109 -0.067405 0 0 0 0 construction
  arc A12 (50.7175, -92.4183) -> (51.9952, -91.6806) centre (35.3606, -64.344) ccw construction
  spline S18 degree 3 poles (51.9952, -91.6806) (51.9804, -91.4564) (51.9582, -91.12) (51.907, -90.6735) (51.8607, -90.3396) (51.8052, -90.0071) (51.7401, -89.6764) (51.6646, -89.3478) (51.578, -89.022) (51.4787, -88.6999) (51.3663, -88.382) (51.2558, -88.1236) (51.1629, -87.9191) (51.1063, -87.7601) (51.0667, -87.596) (51.0484, -87.428) (51.0555, -87.2873) (51.0736, -87.1762) (51.0986, -87.0956) (51.1261, -87.0158) (51.1666, -86.9417) (51.2096, -86.8691) (51.2644, -86.8048) (51.3215, -86.7426) (51.4102, -86.6732) (51.5253, -86.5928) (51.6373, -86.5082) (51.7307, -86.4453) (51.8075, -86.4102) (51.8855, -86.378) (51.9679, -86.3595) (52.0509, -86.3439) (52.1353, -86.3424) (52.2197, -86.3435) (52.3309, -86.3606) (52.4669, -86.3973) (52.6211, -86.4667) (52.7649, -86.5551) (52.8986, -86.658) (53.0644, -86.8096) (53.276, -86.9945) (53.5436, -87.1996) (53.8193, -87.3936) (54.1024, -87.5767) (54.3915, -87.75) (54.686, -87.9141) (54.985, -88.0697) (55.2882, -88.2169) (55.6971, -88.4036) (56.0102, -88.5286) (56.2189, -88.6119) knots -1.0784 -1.0784 -1.0784 -1.0784 -1.010995 -0.977291 -0.943586 -0.909882 -0.876178 -0.842474 -0.80877 -0.775067 -0.741365 -0.707665 -0.690816 -0.67397 -0.657123 -0.640284 -0.623449 -0.615023 -0.606598 -0.598176 -0.589749 -0.581327 -0.572901 -0.564477 -0.556053 -0.5392 -0.522347 -0.513923 -0.505499 -0.497074 -0.488651 -0.480225 -0.471802 -0.463377 -0.454951 -0.438116 -0.421277 -0.40443 -0.387584 -0.370735 -0.337035 -0.303333 -0.26963 -0.235926 -0.202222 -0.168518 -0.134814 -0.101109 -0.067405 0 0 0 0 construction
  arc A13 (56.2189, -88.6119) -> (57.3153, -87.6247) centre (35.3606, -64.344) ccw construction
  spline S19 degree 3 poles (57.3153, -87.6247) (57.2542, -87.4085) (57.1626, -87.084) (57.0196, -86.6579) (56.9049, -86.341) (56.7815, -86.0273) (56.649, -85.7173) (56.5069, -85.4116) (56.3544, -85.111) (56.1903, -84.8165) (56.0143, -84.5289) (55.8525, -84.2992) (55.7191, -84.1184) (55.6307, -83.9746) (55.5579, -83.8224) (55.505, -83.6618) (55.4827, -83.5227) (55.4773, -83.4103) (55.485, -83.3263) (55.4953, -83.2425) (55.5195, -83.1616) (55.5465, -83.0816) (55.5867, -83.0074) (55.6297, -82.9347) (55.702, -82.8484) (55.7978, -82.7458) (55.8898, -82.6398) (55.9681, -82.5588) (56.0359, -82.5085) (56.1055, -82.4607) (56.1823, -82.4255) (56.2602, -82.3931) (56.3425, -82.374) (56.4252, -82.3576) (56.5376, -82.3512) (56.6782, -82.3588) (56.8434, -82.3946) (57.0025, -82.4511) (57.1547, -82.5241) (57.3484, -82.6378) (57.5938, -82.7747) (57.8982, -82.9197) (58.2082, -83.0521) (58.5232, -83.1723) (58.842, -83.2817) (59.1642, -83.3811) (59.489, -83.4711) (59.8162, -83.552) (60.255, -83.6496) (60.5872, -83.7068) (60.8086, -83.7449) knots -1.0784 -1.0784 -1.0784 -1.0784 -1.010995 -0.977291 -0.943586 -0.909882 -0.876178 -0.842474 -0.80877 -0.775067 -0.741365 -0.707665 -0.690816 -0.67397 -0.657123 -0.640284 -0.623449 -0.615023 -0.606598 -0.598176 -0.589749 -0.581327 -0.572901 -0.564477 -0.556053 -0.5392 -0.522347 -0.513923 -0.505499 -0.497074 -0.488651 -0.480225 -0.471802 -0.463377 -0.454951 -0.438116 -0.421277 -0.40443 -0.387584 -0.370735 -0.337035 -0.303333 -0.26963 -0.235926 -0.202222 -0.168518 -0.134814 -0.101109 -0.067405 0 0 0 0 construction
  arc A14 (60.8086, -83.7449) -> (61.6758, -82.5513) centre (35.3606, -64.344) ccw construction
  spline S20 degree 3 poles (61.6758, -82.5513) (61.5711, -82.3525) (61.4141, -82.0542) (61.1857, -81.6671) (61.0076, -81.3809) (60.8216, -81.0998) (60.6276, -80.8241) (60.425, -80.5547) (60.2133, -80.2923) (59.9916, -80.0384) (59.7596, -79.7937) (59.5536, -79.6026) (59.3856, -79.4535) (59.2692, -79.3313) (59.1663, -79.1975) (59.0812, -79.0514) (59.0305, -78.92) (59.0018, -78.8112) (58.9919, -78.7274) (58.9846, -78.6433) (58.9914, -78.5592) (59.0012, -78.4753) (59.025, -78.3943) (59.0519, -78.3143) (59.1048, -78.2148) (59.1772, -78.0945) (59.2451, -77.9717) (59.3049, -77.8762) (59.3607, -77.8129) (59.4189, -77.7517) (59.4867, -77.7013) (59.5561, -77.6534) (59.6326, -77.6176) (59.7101, -77.5843) (59.8187, -77.5547) (59.9579, -77.533) (60.1269, -77.5336) (60.2942, -77.5559) (60.4583, -77.5955) (60.6714, -77.6665) (60.9399, -77.7494) (61.2678, -77.828) (61.5986, -77.893) (61.9316, -77.9451) (62.2663, -77.9858) (62.602, -78.016) (62.9385, -78.0365) (63.2754, -78.0476) (63.7248, -78.0519) (64.0617, -78.0388) (64.2862, -78.03) knots -1.0784 -1.0784 -1.0784 -1.0784 -1.010995 -0.977291 -0.943586 -0.909882 -0.876178 -0.842474 -0.80877 -0.775067 -0.741365 -0.707665 -0.690816 -0.67397 -0.657123 -0.640284 -0.623449 -0.615023 -0.606598 -0.598176 -0.589749 -0.581327 -0.572901 -0.564477 -0.556053 -0.5392 -0.522347 -0.513923 -0.505499 -0.497074 -0.488651 -0.480225 -0.471802 -0.463377 -0.454951 -0.438116 -0.421277 -0.40443 -0.387584 -0.370735 -0.337035 -0.303333 -0.26963 -0.235926 -0.202222 -0.168518 -0.134814 -0.101109 -0.067405 0 0 0 0 construction
  arc A15 (64.2862, -78.03) -> (64.8863, -76.6822) centre (35.3606, -64.344) ccw construction
  spline S21 degree 3 poles (64.8863, -76.6822) (64.7425, -76.5095) (64.5269, -76.2504) (64.223, -75.9192) (63.9893, -75.6763) (63.7489, -75.44) (63.5019, -75.2107) (63.2477, -74.9893) (62.9861, -74.7766) (62.7164, -74.5743) (62.4386, -74.3832) (62.1974, -74.2392) (62.002, -74.1282) (61.8628, -74.0329) (61.7343, -73.9234) (61.6207, -73.7983) (61.5437, -73.6802) (61.4931, -73.5798) (61.466, -73.4999) (61.4413, -73.4191) (61.4305, -73.3354) (61.4226, -73.2513) (61.4291, -73.1671) (61.4388, -73.0833) (61.4698, -72.975) (61.5156, -72.8423) (61.5565, -72.708) (61.5951, -72.6022) (61.6366, -72.5287) (61.6808, -72.4567) (61.7366, -72.3934) (61.7945, -72.332) (61.862, -72.2811) (61.9308, -72.2324) (62.0309, -72.1809) (62.1625, -72.1307) (62.328, -72.0962) (62.4963, -72.0832) (62.665, -72.0879) (62.8882, -72.113) (63.1681, -72.1382) (63.5052, -72.1469) (63.8422, -72.1417) (64.1788, -72.1235) (64.5146, -72.0937) (64.8493, -72.0534) (65.1827, -72.0035) (65.5145, -71.9444) (65.955, -71.8551) (66.2818, -71.7722) (66.4996, -71.717) knots -1.0784 -1.0784 -1.0784 -1.0784 -1.010995 -0.977291 -0.943586 -0.909882 -0.876178 -0.842474 -0.80877 -0.775067 -0.741365 -0.707665 -0.690816 -0.67397 -0.657123 -0.640284 -0.623449 -0.615023 -0.606598 -0.598176 -0.589749 -0.581327 -0.572901 -0.564477 -0.556053 -0.5392 -0.522347 -0.513923 -0.505499 -0.497074 -0.488651 -0.480225 -0.471802 -0.463377 -0.454951 -0.438116 -0.421277 -0.40443 -0.387584 -0.370735 -0.337035 -0.303333 -0.26963 -0.235926 -0.202222 -0.168518 -0.134814 -0.101109 -0.067405 0 0 0 0 construction
  arc A16 (66.4996, -71.717) -> (66.8064, -70.2739) centre (35.3606, -64.344) ccw construction
  spline S22 degree 3 poles (66.8064, -70.2739) (66.6298, -70.1348) (66.365, -69.9262) (65.9989, -69.6655) (65.7198, -69.4764) (65.4356, -69.2952) (65.1462, -69.1223) (64.8515, -68.9586) (64.5515, -68.805) (64.2456, -68.6632) (63.9342, -68.534) (63.6683, -68.4432) (63.4541, -68.3754) (63.2981, -68.311) (63.1496, -68.2307) (63.0125, -68.1319) (62.9127, -68.0324) (62.8422, -67.9447) (62.7991, -67.8722) (62.7582, -67.7983) (62.7302, -67.7187) (62.705, -67.6381) (62.6939, -67.5544) (62.6859, -67.4703) (62.6937, -67.358) (62.711, -67.2187) (62.7231, -67.0788) (62.7388, -66.9673) (62.7641, -66.8867) (62.7923, -66.8072) (62.8338, -66.7336) (62.8777, -66.6615) (62.9331, -66.5977) (62.9903, -66.5358) (63.0775, -66.4646) (63.1958, -66.3881) (63.3504, -66.32) (63.5123, -66.2722) (63.6783, -66.2417) (63.902, -66.2199) (64.1809, -66.1864) (64.5124, -66.1248) (64.8411, -66.0497) (65.1665, -65.9618) (65.4888, -65.8629) (65.8078, -65.7539) (66.1235, -65.6358) (66.4358, -65.5089) (66.8481, -65.33) (67.1505, -65.181) (67.3521, -65.0817) knots -1.0784 -1.0784 -1.0784 -1.0784 -1.010995 -0.977291 -0.943586 -0.909882 -0.876178 -0.842474 -0.80877 -0.775067 -0.741365 -0.707665 -0.690816 -0.67397 -0.657123 -0.640284 -0.623449 -0.615023 -0.606598 -0.598176 -0.589749 -0.581327 -0.572901 -0.564477 -0.556053 -0.5392 -0.522347 -0.513923 -0.505499 -0.497074 -0.488651 -0.480225 -0.471802 -0.463377 -0.454951 -0.438116 -0.421277 -0.40443 -0.387584 -0.370735 -0.337035 -0.303333 -0.26963 -0.235926 -0.202222 -0.168518 -0.134814 -0.101109 -0.067405 0 0 0 0 construction
  arc A17 (67.3521, -65.0817) -> (67.3521, -63.6063) centre (35.3606, -64.344) ccw construction
  spline S23 degree 3 poles (67.3521, -63.6063) (67.1505, -63.507) (66.8481, -63.358) (66.4358, -63.1791) (66.1235, -63.0523) (65.8078, -62.9341) (65.4888, -62.8251) (65.1665, -62.7262) (64.8411, -62.6384) (64.5124, -62.5633) (64.1809, -62.5016) (63.902, -62.4681) (63.6783, -62.4463) (63.5123, -62.4158) (63.3504, -62.3681) (63.1958, -62.2999) (63.0775, -62.2234) (62.9903, -62.1522) (62.9331, -62.0903) (62.8777, -62.0265) (62.8338, -61.9545) (62.7923, -61.8809) (62.7641, -61.8013) (62.7388, -61.7208) (62.7231, -61.6092) (62.711, -61.4694) (62.6937, -61.3301) (62.6859, -61.2177) (62.6939, -61.1337) (62.705, -61.05) (62.7302, -60.9694) (62.7582, -60.8897) (62.7991, -60.8158) (62.8422, -60.7434) (62.9127, -60.6556) (63.0125, -60.5562) (63.1496, -60.4574) (63.2981, -60.377) (63.4541, -60.3127) (63.6683, -60.2448) (63.9342, -60.1541) (64.2456, -60.0249) (64.5515, -59.8831) (64.8515, -59.7294) (65.1462, -59.5657) (65.4356, -59.3928) (65.7198, -59.2116) (65.9989, -59.0226) (66.365, -58.7618) (66.6298, -58.5532) (66.8064, -58.4142) knots -1.0784 -1.0784 -1.0784 -1.0784 -1.010995 -0.977291 -0.943586 -0.909882 -0.876178 -0.842474 -0.80877 -0.775067 -0.741365 -0.707665 -0.690816 -0.67397 -0.657123 -0.640284 -0.623449 -0.615023 -0.606598 -0.598176 -0.589749 -0.581327 -0.572901 -0.564477 -0.556053 -0.5392 -0.522347 -0.513923 -0.505499 -0.497074 -0.488651 -0.480225 -0.471802 -0.463377 -0.454951 -0.438116 -0.421277 -0.40443 -0.387584 -0.370735 -0.337035 -0.303333 -0.26963 -0.235926 -0.202222 -0.168518 -0.134814 -0.101109 -0.067405 0 0 0 0 construction
  arc A18 (66.8064, -58.4142) -> (66.4996, -56.971) centre (35.3606, -64.344) ccw construction
  spline S24 degree 3 poles (66.4996, -56.971) (66.2818, -56.9158) (65.955, -56.833) (65.5145, -56.7437) (65.1827, -56.6845) (64.8493, -56.6346) (64.5146, -56.5943) (64.1788, -56.5646) (63.8422, -56.5463) (63.5052, -56.5412) (63.1681, -56.5498) (62.8882, -56.5751) (62.665, -56.6002) (62.4963, -56.6049) (62.328, -56.5918) (62.1625, -56.5574) (62.0309, -56.5071) (61.9308, -56.4556) (61.862, -56.4069) (61.7945, -56.3561) (61.7366, -56.2947) (61.6808, -56.2313) (61.6366, -56.1594) (61.5951, -56.0858) (61.5565, -55.98) (61.5156, -55.8457) (61.4698, -55.713) (61.4388, -55.6048) (61.4291, -55.5209) (61.4226, -55.4367) (61.4305, -55.3526) (61.4413, -55.2689) (61.466, -55.1881) (61.4931, -55.1083) (61.5437, -55.0078) (61.6207, -54.8898) (61.7343, -54.7646) (61.8628, -54.6552) (62.002, -54.5598) (62.1974, -54.4489) (62.4386, -54.3048) (62.7164, -54.1137) (62.9861, -53.9114) (63.2477, -53.6988) (63.5019, -53.4773) (63.7489, -53.248) (63.9893, -53.0117) (64.223, -52.7688) (64.5269, -52.4376) (64.7425, -52.1785) (64.8863, -52.0058) knots -1.0784 -1.0784 -1.0784 -1.0784 -1.010995 -0.977291 -0.943586 -0.909882 -0.876178 -0.842474 -0.80877 -0.775067 -0.741365 -0.707665 -0.690816 -0.67397 -0.657123 -0.640284 -0.623449 -0.615023 -0.606598 -0.598176 -0.589749 -0.581327 -0.572901 -0.564477 -0.556053 -0.5392 -0.522347 -0.513923 -0.505499 -0.497074 -0.488651 -0.480225 -0.471802 -0.463377 -0.454951 -0.438116 -0.421277 -0.40443 -0.387584 -0.370735 -0.337035 -0.303333 -0.26963 -0.235926 -0.202222 -0.168518 -0.134814 -0.101109 -0.067405 0 0 0 0 construction
  arc A19 (64.8863, -52.0058) -> (64.2862, -50.658) centre (35.3606, -64.344) ccw construction
  spline S25 degree 3 poles (64.2862, -50.658) (64.0617, -50.6493) (63.7248, -50.6361) (63.2754, -50.6404) (62.9385, -50.6515) (62.602, -50.672) (62.2663, -50.7022) (61.9316, -50.7429) (61.5986, -50.795) (61.2678, -50.8601) (60.9399, -50.9386) (60.6714, -51.0215) (60.4583, -51.0925) (60.2942, -51.1322) (60.1269, -51.1544) (59.9579, -51.1551) (59.8187, -51.1333) (59.7101, -51.1037) (59.6326, -51.0704) (59.5561, -51.0347) (59.4867, -50.9867) (59.4189, -50.9363) (59.3607, -50.8751) (59.3049, -50.8118) (59.2451, -50.7163) (59.1772, -50.5935) (59.1048, -50.4732) (59.0519, -50.3738) (59.025, -50.2938) (59.0012, -50.2128) (58.9914, -50.1289) (58.9846, -50.0447) (58.9919, -49.9606) (59.0018, -49.8769) (59.0305, -49.768) (59.0812, -49.6366) (59.1663, -49.4906) (59.2692, -49.3568) (59.3856, -49.2345) (59.5536, -49.0854) (59.7596, -48.8944) (59.9916, -48.6497) (60.2133, -48.3957) (60.425, -48.1333) (60.6276, -47.8639) (60.8216, -47.5882) (61.0076, -47.3071) (61.1857, -47.0209) (61.4141, -46.6338) (61.5711, -46.3355) (61.6758, -46.1367) knots -1.0784 -1.0784 -1.0784 -1.0784 -1.010995 -0.977291 -0.943586 -0.909882 -0.876178 -0.842474 -0.80877 -0.775067 -0.741365 -0.707665 -0.690816 -0.67397 -0.657123 -0.640284 -0.623449 -0.615023 -0.606598 -0.598176 -0.589749 -0.581327 -0.572901 -0.564477 -0.556053 -0.5392 -0.522347 -0.513923 -0.505499 -0.497074 -0.488651 -0.480225 -0.471802 -0.463377 -0.454951 -0.438116 -0.421277 -0.40443 -0.387584 -0.370735 -0.337035 -0.303333 -0.26963 -0.235926 -0.202222 -0.168518 -0.134814 -0.101109 -0.067405 0 0 0 0 construction
  arc A20 (61.6758, -46.1367) -> (60.8086, -44.9431) centre (35.3606, -64.344) ccw construction
  spline S26 degree 3 poles (60.8086, -44.9431) (60.5872, -44.9812) (60.255, -45.0384) (59.8162, -45.1361) (59.489, -45.217) (59.1642, -45.307) (58.842, -45.4063) (58.5232, -45.5157) (58.2082, -45.6359) (57.8982, -45.7683) (57.5938, -45.9133) (57.3484, -46.0502) (57.1547, -46.164) (57.0025, -46.2369) (56.8434, -46.2934) (56.6782, -46.3292) (56.5376, -46.3368) (56.4252, -46.3305) (56.3425, -46.314) (56.2602, -46.295) (56.1823, -46.2625) (56.1055, -46.2273) (56.0359, -46.1795) (55.9681, -46.1292) (55.8898, -46.0483) (55.7978, -45.9422) (55.702, -45.8397) (55.6297, -45.7533) (55.5867, -45.6807) (55.5465, -45.6064) (55.5195, -45.5264) (55.4953, -45.4455) (55.485, -45.3617) (55.4773, -45.2777) (55.4827, -45.1653) (55.505, -45.0262) (55.5579, -44.8657) (55.6307, -44.7134) (55.7191, -44.5696) (55.8525, -44.3888) (56.0143, -44.1591) (56.1903, -43.8715) (56.3544, -43.5771) (56.5069, -43.2764) (56.649, -42.9707) (56.7815, -42.6608) (56.9049, -42.3471) (57.0196, -42.0301) (57.1626, -41.604) (57.2542, -41.2796) (57.3153, -41.0633) knots -1.0784 -1.0784 -1.0784 -1.0784 -1.010995 -0.977291 -0.943586 -0.909882 -0.876178 -0.842474 -0.80877 -0.775067 -0.741365 -0.707665 -0.690816 -0.67397 -0.657123 -0.640284 -0.623449 -0.615023 -0.606598 -0.598176 -0.589749 -0.581327 -0.572901 -0.564477 -0.556053 -0.5392 -0.522347 -0.513923 -0.505499 -0.497074 -0.488651 -0.480225 -0.471802 -0.463377 -0.454951 -0.438116 -0.421277 -0.40443 -0.387584 -0.370735 -0.337035 -0.303333 -0.26963 -0.235926 -0.202222 -0.168518 -0.134814 -0.101109 -0.067405 0 0 0 0 construction
  arc A21 (57.3153, -41.0633) -> (56.2189, -40.0761) centre (35.3606, -64.344) ccw construction
  spline S27 degree 3 poles (56.2189, -40.0761) (56.0102, -40.1594) (55.6971, -40.2845) (55.2882, -40.4712) (54.985, -40.6184) (54.686, -40.7739) (54.3915, -40.9381) (54.1024, -41.1114) (53.8193, -41.2944) (53.5436, -41.4884) (53.276, -41.6935) (53.0644, -41.8784) (52.8986, -42.03) (52.7649, -42.133) (52.6211, -42.2213) (52.4669, -42.2907) (52.3309, -42.3274) (52.2197, -42.3445) (52.1353, -42.3457) (52.0509, -42.3441) (51.9679, -42.3285) (51.8855, -42.3101) (51.8075, -42.2778) (51.7307, -42.2427) (51.6373, -42.1798) (51.5253, -42.0952) (51.4102, -42.0148) (51.3215, -41.9454) (51.2644, -41.8833) (51.2096, -41.819) (51.1666, -41.7463) (51.1261, -41.6722) (51.0986, -41.5924) (51.0736, -41.5119) (51.0555, -41.4008) (51.0484, -41.2601) (51.0667, -41.092) (51.1063, -40.928) (51.1629, -40.769) (51.2558, -40.5644) (51.3663, -40.3061) (51.4787, -39.9882) (51.578, -39.666) (51.6646, -39.3402) (51.7401, -39.0117) (51.8052, -38.6809) (51.8607, -38.3484) (51.907, -38.0146) (51.9582, -37.568) (51.9804, -37.2317) (51.9952, -37.0074) knots -1.0784 -1.0784 -1.0784 -1.0784 -1.010995 -0.977291 -0.943586 -0.909882 -0.876178 -0.842474 -0.80877 -0.775067 -0.741365 -0.707665 -0.690816 -0.67397 -0.657123 -0.640284 -0.623449 -0.615023 -0.606598 -0.598176 -0.589749 -0.581327 -0.572901 -0.564477 -0.556053 -0.5392 -0.522347 -0.513923 -0.505499 -0.497074 -0.488651 -0.480225 -0.471802 -0.463377 -0.454951 -0.438116 -0.421277 -0.40443 -0.387584 -0.370735 -0.337035 -0.303333 -0.26963 -0.235926 -0.202222 -0.168518 -0.134814 -0.101109 -0.067405 0 0 0 0 construction
  arc A22 (51.9952, -37.0074) -> (50.7175, -36.2697) centre (35.3606, -64.344) ccw construction
  spline S28 degree 3 poles (50.7175, -36.2697) (50.5307, -36.3946) (50.2504, -36.582) (49.8893, -36.8497) (49.6233, -37.0567) (49.3632, -37.271) (49.1093, -37.4928) (48.8625, -37.7224) (48.6237, -37.9603) (48.3943, -38.2074) (48.1752, -38.4637) (48.0067, -38.6885) (47.876, -38.8713) (47.7666, -38.9998) (47.6443, -39.1161) (47.508, -39.216) (47.3825, -39.2802) (47.2773, -39.3201) (47.195, -39.3387) (47.1121, -39.3548) (47.0277, -39.3568) (46.9433, -39.3558) (46.8603, -39.3405) (46.7779, -39.3221) (46.6734, -39.28) (46.5463, -39.2206) (46.417, -39.1658) (46.3158, -39.1164) (46.247, -39.0675) (46.1801, -39.016) (46.1229, -38.9539) (46.0679, -38.8898) (46.0243, -38.8175) (45.9831, -38.7439) (45.9424, -38.639) (45.9061, -38.5028) (45.8891, -38.3347) (45.8938, -38.1659) (45.9161, -37.9987) (45.9644, -37.7792) (46.0188, -37.5036) (46.0626, -37.1692) (46.0927, -36.8335) (46.1097, -36.4968) (46.1153, -36.1598) (46.1102, -35.8227) (46.0954, -35.4859) (46.0712, -35.1497) (46.0285, -34.7023) (45.9802, -34.3687) (45.9481, -34.1463) knots -1.0784 -1.0784 -1.0784 -1.0784 -1.010995 -0.977291 -0.943586 -0.909882 -0.876178 -0.842474 -0.80877 -0.775067 -0.741365 -0.707665 -0.690816 -0.67397 -0.657123 -0.640284 -0.623449 -0.615023 -0.606598 -0.598176 -0.589749 -0.581327 -0.572901 -0.564477 -0.556053 -0.5392 -0.522347 -0.513923 -0.505499 -0.497074 -0.488651 -0.480225 -0.471802 -0.463377 -0.454951 -0.438116 -0.421277 -0.40443 -0.387584 -0.370735 -0.337035 -0.303333 -0.26963 -0.235926 -0.202222 -0.168518 -0.134814 -0.101109 -0.067405 0 0 0 0 construction
  arc A23 (45.9481, -34.1463) -> (44.5449, -33.6903) centre (35.3606, -64.344) ccw construction